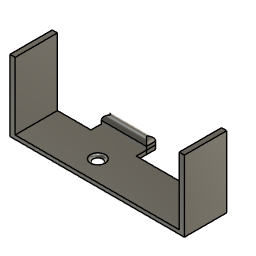
outil_photo v3 (Autodesk Fusion 360 design; units mm, degrees)
Autodesk Fusion 360 part; units mm, degrees
note: some values were not read from the file. Chosen so that the rebuilt part matches the saved one: which pieces of a blend or face edit are solid.
sketch "Esquisse1" plane through (0, 0, 0) normal (0, 0, 1) x (1, 0, 0)
  line L0 (0, 0) -> (127, 0)
  line L1 (127, 0) -> (127, 32.7)
  line L2 (127, 32.7) -> (0, 32.7)
  line L3 (0, 32.7) -> (0, 0)
  circle A0 centre (48, 16) radius 3.75
  line L4 (26, 32.7) -> (61, 32.7)
  line L5 (61, 32.7) -> (61, 47.7)
  line L6 (61, 47.7) -> (26, 47.7)
  line L7 (26, 47.7) -> (26, 32.7)
  line L8 (0, 32.7) -> (-4, 32.7)
  line L9 (-4, 32.7) -> (-4, 0)
  line L10 (-4, 0) -> (0, 0)
  line L11 (0, 0) -> (0, 32.7)
  line L12 (127, 32.7) -> (131, 32.7)
  line L13 (131, 32.7) -> (131, 0)
  line L14 (131, 0) -> (127, 0)
  line L15 (127, 0) -> (127, 32.7)
  dimension "d4" = 127
  dimension "d5" = 32.7
  dimension "d6" = 7.5
  dimension "d7" = 48
  dimension "d8" = 16
  dimension "d9" = 26
  dimension "d10" = 35
  dimension "d11" = 15
  dimension "d13" = 4
  dimension "d14" = 4
  constraint horizontal L0
  constraint vertical L1
  constraint horizontal L2
  constraint vertical L3
  constraint coincident L0.start L3.end
  constraint horizontal L4
  constraint vertical L5
  constraint horizontal L6
  constraint vertical L7
  constraint coincident L2 L4.start
  constraint horizontal L8
  constraint vertical L9
  constraint horizontal L10
  constraint vertical L11
  constraint horizontal L12
  constraint vertical L13
  constraint horizontal L14
  constraint vertical L15
  constraint collinear L0 L10
  constraint collinear L0 L14
  measures "d4" distance of L0.start L0.end
  measures "d5" distance of L0.start L2.end
  measures "d6" diameter of A0
  measures "d7" distance of L3 A0.centre
  measures "d8" distance of L0 A0.centre
  measures "d9" distance of L3 L7
  measures "d10" distance of L5 L7
  measures "d11" distance of L4 L6
  measures "d13" distance of L2.end L8.end
  measures "d14" distance of L1.end L12.end
extrude "Extrusion1" add sketch "Esquisse1" along normal blind 25 contours L3 L8 L9 L10 L11 | L1 L12 L13 L14 L15 makes body 1 at (-4, 21.8, 8.3333) makes body 2 at (127, 10.9, 8.3333)
extrude "Extrusion2" add sketch "Esquisse1" along normal blind 3 contours L0 L1 L2 L3 L4 L11 L15 bodies 1 2
extrude "Extrusion3" add sketch "Esquisse1" along normal blind 3 contours L2 L4 L5 L6 L7 bodies 1
extrude "Extrusion4" cut 1 faces at (-1.3333, 10.9, 25) along direction (0, 0, -1) blind 25 on bodies 1 bodies 1
extrude "Extrusion5" cut 1 faces at (129.6667, 21.8, 25) along direction (0, 0, -1) blind 25 on bodies 1 bodies 1
extrude "Extrusion6" add sketch "Esquisse1" along normal blind 55 contours L3 L8 L9 L10 L11 | L1 L12 L13 L14 L15 bodies 1
extrude "Extrusion7" add sketch "Esquisse1" along normal blind 12 separate body contours L2 L4 L5 L6 L7 makes body 3
extrude "Extrusion8" cut 1 faces at (49.3333, 32.7, 4) along direction (0, 1, 0) blind 8 on bodies 3 bodies 3
extrude "Extrusion9" cut 1 faces at (37.6667, 43.0333, 12) along direction (0, 0, -1) blind 3 on bodies 3 bodies 3
fillet "Congé1" radius 3.5 4 edges at (61, 44.2, 9) (43.5, 40.7, 9) (43.5, 47.7, 9) (26, 44.2, 9) on bodies 3
fillet "Congé2" radius 2 2 edges at (44.5038, 17.3561, 3) (44.5038, 17.3561, 0) on bodies 1
equation "longueur_appareille = 127 mm"
equation "largeur_appareil = 32.7 mm"
equation "hauteur_appareil_G = 71.5 mm"
equation "d4 = longueur_appareille"
equation "d5 = largeur_appareil"
equation "epaisseur = 4 mm"
equation "d13 = epaisseur"
equation "d14 = epaisseur"
